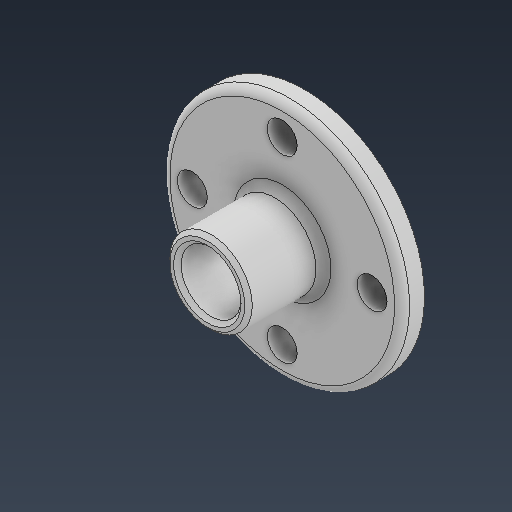
# Autodesk Inventor part: МУФТА НА ВАЛ бол
Saved by Autodesk Inventor 2026 (Build 300175000, 175)
## iProperties
Created: 2026-01-10
Part Number: МУФТА НА ВАЛ бол
Material: Типовые
Document SubType Name: Modeling
Designer: GameHD
Density: 1 g/cm^3
Appearance: По умолчанию
Author: GameHD
Autodesk Inventor part; units mm, degrees
ref_plane "YZ Plane" through (0, 0, 0) normal (1, 0, 0) x (0, 1, 0)
ref_plane "XZ Plane" through (0, 0, 0) normal (0, 1, 0) x (-1, 0, 0)
ref_plane "XY Plane" through (0, 0, 0) normal (0, 0, 1) x (1, 0, 0)
sketch "Эскиз1" plane through (0, 0, 0) normal (0, 0, 1) x (1, 0, 0)
  circle A0 centre (0, 0) radius 16
  circle A1 centre (0, 0) radius 12
  circle A2 centre (-12, 0) radius 2
  circle A3 centre (0, -12) radius 2
  circle A4 centre (12, 0) radius 2
  circle A5 centre (0, 12) radius 2
  circle A6 centre (0, 0) radius 4
  dimension "d1" = 24
  dimension "d0" = 32
  dimension "d2" = 4
  dimension "d5" = 360
  dimension "d7" = 8
  constraints: 6 centre point, 5 coincident, 1 horizontal alignment, 11 other
  measures "d0" diameter of A0
  measures "d2" diameter of A2
  measures "d7" diameter of A6
extrude "Выдавливание1" add sketch "Эскиз1" along normal blind 3 contours A0 | A4 A1 A3 A2 A5
sketch "Эскиз2" plane through (0, 0, 3) normal (0, 0, 1) x (1, 0, 0)
  circle A0 centre (0, 0) radius 5.5
  circle A1 centre (0, 0) radius 16 projected
  circle A2 centre (0, 12) radius 2 projected
  circle A3 centre (-12, 0) radius 2 projected
  circle A4 centre (0, -12) radius 2 projected
  circle A5 centre (0, 0) radius 4 projected
  circle A6 centre (12, 0) radius 2 projected
  dimension "d10" = 11
  constraints: 1 centre point, 1 coincident
  measures "d10" diameter of A0
extrude "Выдавливание2" add sketch "Эскиз2" along normal blind 10 contours A0
fillet "Сопряжение1" radius 1 2 edges at (-16, 0, 3) (-5.5, 0, 3)
chamfer "Фаска1" distance 0.5 angle 45 2 edges at (-5.5, 0, 13) (-4, 0, 13)
